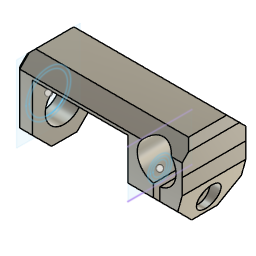
PARKING_LIGHT_HOLDER (Autodesk Fusion 360 design; units mm, degrees)
Autodesk Fusion 360 part; units mm, degrees
sketch "Esquisse1" plane through (0, 0, 0) normal (0, 1, 0) x (1, 0, 0)
  circle A0 centre (0, 0) radius 6.1 construction
  line L0 (8, 0) -> (8, 16) construction
  line L1 (-9, 0.0178) -> (-9, 15)
  line L2 (-8, 16) -> (8, 16) construction
  line L3 (1, 0) -> (-1, 0)
  line L4 (-1, 0) -> (-1, 16) construction
  line L5 (-1, 16) -> (1, 16) construction
  line L6 (1, 16) -> (1, 0) construction
  line L7 (8, 0) -> (-9, 0) construction
  line L8 (8, -6) -> (8, 0)
  line L9 (8, 5) -> (5, 16)
  arc A1 (-1, 6.0175) -> (1, 6.0175) centre (0, 0) ccw
  line L10 (1, 16) -> (1, 6.0175)
  line L11 (1, 16) -> (5, 16)
  line L12 (-1, 6.0175) -> (-1, 16)
  line L13 (-1, 16) -> (-9, 16)
  line L14 (8, 5) -> (8, 0)
  line L15 (-39, -3) -> (-39, 18)
  line L16 (-39, 18) -> (-44, 18)
  line L17 (-44, 18) -> (-44, -6)
  line L18 (-39, -3) -> (-9, -3.0001)
  line L19 (-9, -3.0001) -> (-9, 0.0178)
  line L20 (6, -8) -> (-42, -8)
  line L21 (8, -6) -> (6, -8)
  line L22 (-44, -6) -> (-42, -8)
  line L23 (-8, 16) -> (-9, 15)
  point P0 (8, -8)
  point P1 (-44, -8)
  dimension "d1" = 12.2
  dimension "d4" = 16
  dimension "d5" = 8
  dimension "d6" = 2
  dimension "d7" = 1
  dimension "d44" = 21
  dimension "d46" = 30
  dimension "d47" = 5
  dimension "d48" = 9
  dimension "d49" = 2
  dimension "d50" = 2
  dimension "d51" = 2
  dimension "d52" = 2
  dimension "d53" = 1
  dimension "d54" = 1
  constraint coincident A0.centre A1.centre
  constraint vertical L0
  constraint vertical L1
  constraint perpendicular L0 L2
  constraint horizontal L3
  constraint vertical L4
  constraint vertical L6
  constraint coincident L2 L4.end
  constraint horizontal L7
  constraint vertical L8
  constraint coincident L0 L9.start
  constraint coincident L6 A1.end
  constraint coincident A0 A1.start
  constraint coincident L4 A1.start
  constraint vertical L15
  constraint perpendicular L15 L16
  constraint perpendicular L16 L17
  constraint coincident P0 L8
  constraint coincident P0 L20
  constraint coincident P1 L17
  constraint coincident P1 L20
  constraint coincident L13.end L2
  constraint coincident L13.end L1
  measures "d1" diameter of A0
  measures "d4" distance of A0.centre L2
  measures "d5" distance of A0.centre L0
  measures "d6" distance of L4 L6
  measures "d7" distance of A0.centre L4
  measures "d44" distance of L15.start L15.end
  measures "d46" distance of L1 L15
  measures "d47" distance of L15.end L16.end
  measures "d48" distance of L1 A0.centre
  measures "d49" distance of P0 L8.start
  measures "d50" distance of P0 L20.start
  measures "d51" distance of P1 L17.end
  measures "d52" distance of P1 L20.end
  measures "d53" distance of L13.end L2.start
  measures "d54" distance of L13.end L1.end
extrude "Extrusion1" add sketch "Esquisse1" along normal blind 20
sketch "Esquisse3" plane through (-9, 0, 0) normal (-1, 0, 0) x (0, -1, 0)
  line L0 (0, -15) -> (0, -0.0178)
  line L1 (-20, -0.0178) -> (-20, -15)
  circle A0 centre (-10, -11) radius 2.95
  circle A1 centre (-10, -11) radius 2.15
  circle A2 centre (-10, -11) radius 3.75
  line L2 (0, -0.0178) -> (-20, -0.0178)
  line L3 (-20, -15) -> (0, -15)
  dimension "d24" = 5.9
  dimension "d26" = 4.3
  dimension "d27" = 7.5
  constraint concentric A0 A1
  constraint concentric A1 A2
  measures "d24" diameter of A0
  measures "d26" diameter of A1
  measures "d27" diameter of A2
extrude "Extrusion5" cut sketch "Esquisse3" against normal blind 20 contours A1
extrude "Extrusion6" cut sketch "Esquisse3" against normal blind 10 from surface at -12 contours A0 | A2
extrude "Extrusion7" cut sketch "Esquisse3" against normal blind 9 contours A0
sketch "Esquisse4" plane through (-9, 0, 0) normal (-1, 0, 0) x (0, -1, 0)
  line L0 (-20, -16) -> (0, -16)
  line L1 (-20, -16) -> (-20, -10)
  line L2 (-20, -16) -> (-14, -16)
  line L3 (-14, -16) -> (-20, -10)
  line L4 (0, -16) -> (0, -10)
  line L5 (0, -16) -> (0, -10)
  line L6 (0, -16) -> (-6, -16)
  line L7 (0, -10) -> (-6, -16)
  point P0 (0, -15)
  point P1 (-20, -15)
  dimension "d39" = 6
  dimension "d40" = 6
  dimension "d56" = 6
  dimension "d57" = 6
  constraint coincident L0.start L1.start
  constraint perpendicular L0 L1
  constraint perpendicular L1 L2
  constraint coincident L0.end L4.start
  constraint perpendicular L0 L4
  constraint perpendicular L0 L5
  constraint perpendicular L4 L6
  measures "d39" distance of L0.start L1.end
  measures "d40" distance of L0.start L2.end
  measures "d56" distance of L0.end L4.end
  measures "d57" distance of L0.end L6.end
extrude "Extrusion8" cut sketch "Esquisse4" along normal up to surface end surface through (8, 0, -5) normal (0.964764, 0, -0.263117) offset 0
sketch "Esquisse5" plane through (-44, 0, 0) normal (-1, 0, 0) x (0, -1, 0)
  line L0 (0, -18) -> (0, 6)
  line L1 (0, 6) -> (-20, 6)
  line L2 (-20, 6) -> (-20, -18)
  line L3 (-20, -18) -> (0, -18)
  circle A0 centre (-10, -8) radius 6
  circle A1 centre (-10, -8) radius 7
  dimension "d58" = 12
  dimension "d59" = 10
  dimension "d62" = 14
  constraint concentric A0 A1
  measures "d58" diameter of A0
  measures "d59" distance of L3 A0.centre
  measures "d62" diameter of A1
extrude "Extrusion9" cut sketch "Esquisse5" against normal blind 5 contours A0
extrude "Extrusion10" add sketch "Esquisse5" along normal blind 2 contours A1
chamfer "Chanfrein1" distance 6 angle 45 2 edges at (-41.5, 20, -18) (-41.5, 0, -18)
chamfer "Chanfrein2" distance 4 angle 45 2 edges at (-18, 0, 8) (-18, 20, 8)
chamfer "Chanfrein3" distance 1 angle 45 7 edges at (-44, 20, -4) (-44, 17, -15) (-44, 10, -18) (-44, 3, -15) (-44, 0, -4) (-44, 1, 5) (-44, 19, 5)
equation "d50 = d49"
equation "d52 = d51"
equation "d54 = d53"
